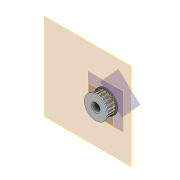
# Autodesk Inventor part: 00_XYTable_pulley_M3
Saved by Autodesk Inventor 2022 (Build 260153000, 153)
## iProperties
Created: 2021-12-06
Part Number: 00_XYTable_pulley_M3
Material: Generisch
Document SubType Name: Modeling
Designer: diederichbenedict
Density: 1 g/cm^3
Appearance: Vorgabe
Author: diederichbenedict
Autodesk Inventor part; units mm, degrees
ref_plane "YZ Plane" through (0, 0, 0) normal (1, 0, 0) x (0, 1, 0)
ref_plane "XZ Plane" through (0, 0, 0) normal (0, 1, 0) x (-1, 0, 0)
ref_plane "XY Plane" through (0, 0, 0) normal (0, 0, 1) x (1, 0, 0)
ref_plane "Arbeitsebene1" through (9.0446, -5.9844, -8.9339) normal (-0.0000016, 0.0000014, -1) x (0.6719093, 0.7406335, 0)
ref_plane "Arbeitsebene2" through (0, 0, 0) normal (0, 0, 1) x (1, 0, 0)
sketch "Skizze1" plane through (0, 0, 0) normal (0, 0, 1) x (1, 0, 0)
  line L0 (9.0319, -5.0529) -> (8.5778, -4.8487) projected
  line L1 (9.0319, -5.0529) -> (9.0446, -5.9844) projected
  circle A0 centre (11.0313, -0.0002) radius 6.3053 projected
  line L2 (7.8724, -5.4572) -> (8.5778, -4.8487) projected
  line L3 (9.0424, -5.9926) -> (9.7112, -6.1745) projected
  line L4 (10.1962, -5.3696) -> (9.7134, -6.1663) projected
  line L5 (10.6911, -5.4235) -> (10.1962, -5.3696) projected
  line L6 (10.6911, -5.4235) -> (10.9911, -6.3054) projected
  circle A1 centre (11.0313, -0.0002) radius 5.4339
  line L7 (9.0319, -5.0529) -> (9.0424, -5.9926)
  line L8 (9.7112, -6.1745) -> (10.1962, -5.3696)
  circle A2 centre (11.0313, -0.0002) radius 2.25 projected
  point P0 (0, 0)
  point P1 (8.5779, -4.8487)
  point P2 (9.2649, -6.0531)
  point P3 (9.4887, -6.114)
  constraints: 4 end point, 4 other
extrude "Extrusion1" add sketch "Skizze1" along normal blind 5.5 contours A1 L4 A0 L1 | L0 A1 L5
pattern_circular "Runde Anordnung1" count 20 over 360 about axis through (11.0313, -0.0002, 0) along (0, 0, 1) of "Extrusion1"
sketch "Skizze2" plane through (0, 0, 5.5) normal (0, 0, 1) x (1, 0, 0)
  line L0 (9.0319, -5.0529) -> (9.0446, -5.9844) projected
  arc A0 (9.0446, -5.9844) -> (9.2649, -6.0531) centre (11.0313, -0.0002) ccw projected
  line L1 (9.2649, -6.0531) -> (9.4887, -6.114) projected
  arc A1 (9.4887, -6.114) -> (9.7134, -6.1663) centre (11.0313, -0.0002) ccw projected
  line L2 (9.7134, -6.1663) -> (10.1962, -5.3696) projected
  arc A2 (11.8963, -5.3648) -> (12.3836, -5.2631) centre (11.0313, -0.0002) ccw projected
  circle A3 centre (11.0313, -0.0002) radius 7
  arc A4 (10.1962, -5.3696) -> (10.6911, -5.4235) centre (11.0313, -0.0002) ccw projected
  line L3 (10.6911, -5.4235) -> (10.9911, -6.3054) projected
  arc A5 (10.9911, -6.3054) -> (11.2218, -6.3027) centre (11.0313, -0.0002) ccw projected
  line L4 (11.2218, -6.3027) -> (11.4535, -6.2914) projected
  arc A6 (11.4535, -6.2914) -> (11.6833, -6.2717) centre (11.0313, -0.0002) ccw projected
  line L5 (11.6833, -6.2717) -> (11.8963, -5.3648) projected
  line L6 (12.3836, -5.2631) -> (12.9415, -6.0092) projected
  arc A7 (12.9415, -6.0092) -> (13.1601, -5.9353) centre (11.0313, -0.0002) ccw projected
  line L7 (13.1601, -5.9353) -> (13.3769, -5.853) projected
  arc A8 (13.3769, -5.853) -> (13.5894, -5.7633) centre (11.0313, -0.0002) ccw projected
  line L8 (13.5894, -5.7633) -> (13.5117, -4.8349) projected
  arc A9 (13.5117, -4.8349) -> (13.9438, -4.5877) centre (11.0313, -0.0002) ccw projected
  line L9 (13.9438, -4.5877) -> (14.7049, -5.1249) projected
  arc A10 (14.7049, -5.1249) -> (14.8899, -4.987) centre (11.0313, -0.0002) ccw projected
  line L10 (14.8899, -4.987) -> (15.0707, -4.8417) projected
  arc A11 (15.0707, -4.8417) -> (15.2451, -4.6907) centre (11.0313, -0.0002) ccw projected
  line L11 (15.2451, -4.6907) -> (14.8843, -3.8318) projected
  arc A12 (14.8843, -3.8318) -> (15.2188, -3.4631) centre (11.0313, -0.0002) ccw projected
  line L12 (15.2188, -3.4631) -> (16.1087, -3.7388) projected
  arc A13 (16.1087, -3.7388) -> (16.2421, -3.5506) centre (11.0313, -0.0002) ccw projected
  line L13 (16.2421, -3.5506) -> (16.3691, -3.3565) projected
  arc A14 (16.3691, -3.3565) -> (16.4883, -3.159) centre (11.0313, -0.0002) ccw projected
  line L14 (16.4883, -3.159) -> (15.8798, -2.4536) projected
  arc A15 (15.8798, -2.4536) -> (16.0839, -1.9996) centre (11.0313, -0.0002) ccw projected
  line L15 (16.0839, -1.9996) -> (17.0155, -1.9869) projected
  arc A16 (17.0155, -1.9869) -> (17.0841, -1.7666) centre (11.0313, -0.0002) ccw projected
  line L16 (17.0841, -1.7666) -> (17.145, -1.5428) projected
  arc A17 (17.145, -1.5428) -> (17.1973, -1.3181) centre (11.0313, -0.0002) ccw projected
  line L17 (17.1973, -1.3181) -> (16.4006, -0.8353) projected
  arc A18 (16.4006, -0.8353) -> (16.4545, -0.3404) centre (11.0313, -0.0002) ccw projected
  line L18 (16.4545, -0.3404) -> (17.3365, -0.0404) projected
  arc A19 (17.3365, -0.0404) -> (17.3337, 0.1903) centre (11.0313, -0.0002) ccw projected
  line L19 (17.3337, 0.1903) -> (17.3224, 0.422) projected
  arc A20 (17.3224, 0.422) -> (17.3028, 0.6518) centre (11.0313, -0.0002) ccw projected
  line L20 (17.3028, 0.6518) -> (16.3959, 0.8648) projected
  arc A21 (16.3959, 0.8648) -> (16.2942, 1.3521) centre (11.0313, -0.0002) ccw projected
  line L21 (16.2942, 1.3521) -> (17.0403, 1.91) projected
  arc A22 (17.0403, 1.91) -> (16.9664, 2.1286) centre (11.0313, -0.0002) ccw projected
  line L22 (16.9664, 2.1286) -> (16.8841, 2.3454) projected
  arc A23 (16.8841, 2.3454) -> (16.7943, 2.5579) centre (11.0313, -0.0002) ccw projected
  line L23 (16.7943, 2.5579) -> (15.866, 2.4802) projected
  arc A24 (15.866, 2.4802) -> (15.6187, 2.9123) centre (11.0313, -0.0002) ccw projected
  line L24 (15.6187, 2.9123) -> (16.1559, 3.6734) projected
  arc A25 (16.1559, 3.6734) -> (16.0181, 3.8584) centre (11.0313, -0.0002) ccw projected
  line L25 (16.0181, 3.8584) -> (15.8728, 4.0392) projected
  arc A26 (15.8728, 4.0392) -> (15.7218, 4.2136) centre (11.0313, -0.0002) ccw projected
  line L26 (15.7218, 4.2136) -> (14.8629, 3.8528) projected
  arc A27 (14.8629, 3.8528) -> (14.4942, 4.1873) centre (11.0313, -0.0002) ccw projected
  line L27 (14.4942, 4.1873) -> (14.7699, 5.0772) projected
  arc A28 (14.7699, 5.0772) -> (14.5816, 5.2106) centre (11.0313, -0.0002) ccw projected
  line L28 (14.5816, 5.2106) -> (14.3876, 5.3376) projected
  arc A29 (14.3876, 5.3376) -> (14.19, 5.4568) centre (11.0313, -0.0002) ccw projected
  line L29 (14.19, 5.4568) -> (13.4847, 4.8483) projected
  arc A30 (13.4847, 4.8483) -> (13.0307, 5.0524) centre (11.0313, -0.0002) ccw projected
  line L30 (13.0307, 5.0524) -> (13.0179, 5.984) projected
  arc A31 (13.0179, 5.984) -> (12.7976, 6.0526) centre (11.0313, -0.0002) ccw projected
  line L31 (12.7976, 6.0526) -> (12.5738, 6.1135) projected
  arc A32 (12.5738, 6.1135) -> (12.3491, 6.1658) centre (11.0313, -0.0002) ccw projected
  line L32 (12.3491, 6.1658) -> (11.8663, 5.3691) projected
  arc A33 (11.8663, 5.3691) -> (11.3715, 5.423) centre (11.0313, -0.0002) ccw projected
  line L33 (11.3715, 5.423) -> (11.0715, 6.305) projected
  arc A34 (11.0715, 6.305) -> (10.8407, 6.3022) centre (11.0313, -0.0002) ccw projected
  line L34 (10.8407, 6.3022) -> (10.6091, 6.2909) projected
  arc A35 (10.6091, 6.2909) -> (10.3792, 6.2713) centre (11.0313, -0.0002) ccw projected
  line L35 (10.3792, 6.2713) -> (10.1662, 5.3644) projected
  arc A36 (10.1662, 5.3644) -> (9.6789, 5.2627) centre (11.0313, -0.0002) ccw projected
  line L36 (9.6789, 5.2627) -> (9.1211, 6.0088) projected
  arc A37 (9.1211, 6.0088) -> (8.9025, 5.9349) centre (11.0313, -0.0002) ccw projected
  line L37 (8.9025, 5.9349) -> (8.6857, 5.8526) projected
  arc A38 (8.6857, 5.8526) -> (8.4731, 5.7628) centre (11.0313, -0.0002) ccw projected
  line L38 (8.4731, 5.7628) -> (8.5508, 4.8345) projected
  arc A39 (8.5508, 4.8345) -> (8.1188, 4.5872) centre (11.0313, -0.0002) ccw projected
  line L39 (8.1188, 4.5872) -> (7.3577, 5.1244) projected
  arc A40 (7.3577, 5.1244) -> (7.1726, 4.9866) centre (11.0313, -0.0002) ccw projected
  line L40 (7.1726, 4.9866) -> (6.9919, 4.8413) projected
  arc A41 (6.9919, 4.8413) -> (6.8174, 4.6903) centre (11.0313, -0.0002) ccw projected
  line L41 (6.8174, 4.6903) -> (7.1782, 3.8314) projected
  arc A42 (7.1782, 3.8314) -> (6.8437, 3.4627) centre (11.0313, -0.0002) ccw projected
  line L42 (6.8437, 3.4627) -> (5.9539, 3.7384) projected
  arc A43 (5.9539, 3.7384) -> (5.8205, 3.5501) centre (11.0313, -0.0002) ccw projected
  line L43 (5.8205, 3.5501) -> (5.6934, 3.3561) projected
  arc A44 (5.6934, 3.3561) -> (5.5742, 3.1585) centre (11.0313, -0.0002) ccw projected
  line L44 (5.5742, 3.1585) -> (6.1828, 2.4532) projected
  arc A45 (6.1828, 2.4532) -> (5.9786, 1.9992) centre (11.0313, -0.0002) ccw projected
  line L45 (5.9786, 1.9992) -> (5.0471, 1.9864) projected
  arc A46 (5.0471, 1.9864) -> (4.9784, 1.7661) centre (11.0313, -0.0002) ccw projected
  line L46 (4.9784, 1.7661) -> (4.9175, 1.5423) projected
  arc A47 (4.9175, 1.5423) -> (4.8652, 1.3176) centre (11.0313, -0.0002) ccw projected
  line L47 (4.8652, 1.3176) -> (5.6619, 0.8348) projected
  arc A48 (5.6619, 0.8348) -> (5.608, 0.34) centre (11.0313, -0.0002) ccw projected
  line L48 (5.608, 0.34) -> (4.7261, 0.04) projected
  arc A49 (4.7261, 0.04) -> (4.7288, -0.1908) centre (11.0313, -0.0002) ccw projected
  line L49 (4.7288, -0.1908) -> (4.7401, -0.4224) projected
  arc A50 (4.7401, -0.4224) -> (4.7598, -0.6523) centre (11.0313, -0.0002) ccw projected
  line L50 (4.7598, -0.6523) -> (5.6667, -0.8653) projected
  arc A51 (5.6667, -0.8653) -> (5.7684, -1.3526) centre (11.0313, -0.0002) ccw projected
  line L51 (5.7684, -1.3526) -> (5.0223, -1.9104) projected
  arc A52 (5.0223, -1.9104) -> (5.0962, -2.129) centre (11.0313, -0.0002) ccw projected
  line L52 (5.0962, -2.129) -> (5.1785, -2.3458) projected
  arc A53 (5.1785, -2.3458) -> (5.2682, -2.5584) centre (11.0313, -0.0002) ccw projected
  line L53 (5.2682, -2.5584) -> (6.1966, -2.4807) projected
  arc A54 (6.1966, -2.4807) -> (6.4438, -2.9127) centre (11.0313, -0.0002) ccw projected
  line L54 (6.4438, -2.9127) -> (5.9066, -3.6738) projected
  arc A55 (5.9066, -3.6738) -> (6.0445, -3.8589) centre (11.0313, -0.0002) ccw projected
  line L55 (6.0445, -3.8589) -> (6.1898, -4.0396) projected
  arc A56 (6.1898, -4.0396) -> (6.3408, -4.2141) centre (11.0313, -0.0002) ccw projected
  line L56 (6.3408, -4.2141) -> (7.1997, -3.8533) projected
  arc A57 (7.1997, -3.8533) -> (7.5684, -4.1878) centre (11.0313, -0.0002) ccw projected
  line L57 (7.5684, -4.1878) -> (7.2927, -5.0776) projected
  arc A58 (7.2927, -5.0776) -> (7.4809, -5.211) centre (11.0313, -0.0002) ccw projected
  line L58 (7.4809, -5.211) -> (7.675, -5.3381) projected
  arc A59 (7.675, -5.3381) -> (7.8725, -5.4573) centre (11.0313, -0.0002) ccw projected
  line L59 (7.8725, -5.4573) -> (8.5779, -4.8487) projected
  arc A60 (8.5779, -4.8487) -> (9.0319, -5.0529) centre (11.0313, -0.0002) ccw projected
  circle A61 centre (11.0313, -0.0002) radius 2.25 projected
  point P0 (0, 0)
  dimension "d6" = 14
  constraints: 1 centre point
  measures "d6" diameter of A3
extrude "Extrusion2" add sketch "Skizze2" along normal blind 0.6 contours A60 L59 A59 L58 A58 L57 A57 L56 A56 L55 A55 L54 A54 L53 A53 L52 A52 L51 A51 L50 A50 L49 A49 L48 A48 L47 A47 L46 A46 L45 A45 L44 A44 L43 A43 L42 A42 L41 A41 L40 A40 L39 A39 L38 A38 L37 A37 L36 A36 L35 A35 L34 A34 L33 A33 L32 A32 L31 A31 L30 A30 L29 A29 L28 A28 L27 A27 L26 A26 L25 A25 L24 A24 L23 A23 L22 A22 L21 A21 L20 A20 L19 A19 L18 A18 L17 A17 L16 A16 L15 A15 L14 A14 L13 A13 L12 A12 L11 A11 L10 A10 L9 A9 L8 A8 L7 A7 L6 A2 L5 A6 L4 A5 L3 A4 L2 A1 L1 A0 L0 | A3
ref_plane "Arbeitsebene3" through (11.0313, -0.0002, 3.05) normal (0, 0, 1) x (1, 0, 0)
ref_plane "Arbeitsebene4" through (11.0313, -0.0002, 0) normal (0, 0, -1) x (-1, 0, 0)
sketch "Skizze5" plane through (11.0313, -0.0002, 0) normal (0, 0, -1) x (-1, 0, 0)
  circle A0 centre (0, 0) radius 7 projected
  circle A1 centre (0, 0) radius 2.205
  circle A2 centre (0, 0) radius 2.25 projected
  circle A3 centre (0, 0) radius 2.45
  circle A4 centre (0, 0) radius 2
  point P0 (11.0313, 0.0002)
  dimension "d12" = 4.9
  dimension "d13" = 4
  constraints: 3 centre point, 3 coincident
  measures "d12" diameter of A3
  measures "d13" diameter of A4
extrude "Extrusion4" add sketch "Skizze5" along normal blind 2 contours A1 | A2 | A3
sketch "Skizze6" plane through (0, 0, 0) normal (0, 0, -1) x (-1, 0, 0)
  circle A0 centre (-11.0313, -0.0002) radius 7 projected
  circle A1 centre (-11.0313, -0.0002) radius 2 projected
  point P0 (0, 0)
extrude "Extrusion5" add sketch "Skizze6" along normal blind 0.5
sketch "Skizze7" plane through (11.0313, -0.0002, -0.5) normal (0, 0, -1) x (-1, 0, 0)
  circle A0 centre (0, 0) radius 2.45 projected
  circle A1 centre (0, 0) radius 2.95
  point P0 (11.0313, 0.0002)
  dimension "d18" = 0.5
  constraints: 1 centre point
  measures "d18" radial gap between concentric circles of A0 A1
extrude "Extrusion6" add sketch "Skizze7" along normal blind 0.3
chamfer "Fase1" distance 0.5 angle 45 1 edges at (8.7813, -0.0002, 6.1)
